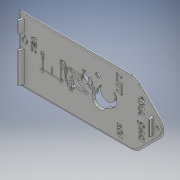
# Autodesk Inventor part: DynamicClampTopCompact
Saved by Autodesk Inventor 2017 (Build 210142000, 142)
## iProperties
Created: 2016-10-04
Part Number: DynamicClampTopCompact
Material: Generic
Document SubType Name: Modeling
Designer: andrew
Density: 1 g/cm^3
Appearance: Default
Author: andrew
Autodesk Inventor part; units mm, degrees
(part 1 of 2)
ref_plane "YZ Plane" through (0, 0, 0) normal (1, 0, 0) x (0, 1, 0)
ref_plane "XZ Plane" through (0, 0, 0) normal (0, 1, 0) x (-1, 0, 0)
ref_plane "XY Plane" through (0, 0, 0) normal (0, 0, 1) x (1, 0, 0)
sketch "Sketch1" plane through (0, 0, 0) normal (0, 1, 0) x (-1, 0, 0)
  line L0 (70.1002, -51.1999) -> (70.1002, -37.9894) construction
  line L1 (70.1002, -37.9894) -> (68.1002, -37.9894) construction
  line L2 (68.1002, -37.9894) -> (68.1002, -48.1999) construction
  arc A0 (67.1002, -49.1999) -> (68.1002, -48.1999) centre (67.1002, -48.1999) ccw construction
  arc A1 (10.6644, -48.6141) -> (12.0787, -49.1999) centre (12.0787, -47.1999) ccw construction
  line L3 (10.6644, -48.6141) -> (10.336, -48.2857) construction
  arc A2 (10.336, -48.2857) -> (8.9218, -47.6999) centre (8.9218, -49.6999) ccw construction
  line L4 (8.9218, -47.6999) -> (-17.9958, -47.6999) construction
  arc A3 (-24.0062, -45.2103) -> (-17.9958, -47.6999) centre (-17.9958, -39.1999) ccw construction
  line L5 (-24.0062, -45.2103) -> (-44.1562, -25.0603) construction
  arc A4 (-44.1562, -13.0395) -> (-44.1562, -25.0603) centre (-38.1458, -19.0499) ccw construction
  line L6 (-44.1562, -13.0395) -> (-24.0062, 7.1105) construction
  arc A5 (-17.9958, 9.6001) -> (-24.0062, 7.1105) centre (-17.9958, 1.1001) ccw construction
  line L7 (-17.9958, 9.6001) -> (8.9218, 9.6001) construction
  arc A6 (8.9218, 9.6001) -> (10.336, 10.1859) centre (8.9218, 11.6001) ccw construction
  line L8 (10.336, 10.1859) -> (10.6644, 10.5143) construction
  arc A7 (12.0787, 11.1001) -> (10.6644, 10.5143) centre (12.0787, 9.1001) ccw construction
  arc A8 (68.1002, 10.1001) -> (67.1002, 11.1001) centre (67.1002, 10.1001) ccw construction
  line L9 (68.1002, 10.1001) -> (68.1002, 5.7045) construction
  line L10 (68.1002, 5.7045) -> (70.1002, 5.7045) construction
  line L11 (70.1002, 5.7045) -> (70.1002, 13.1001) construction
  arc A9 (-17.9958, 13.1001) -> (-26.4811, 9.5854) centre (-17.9958, 1.1001) ccw construction
  line L12 (-26.4811, 9.5854) -> (-46.6311, -10.5646) construction
  arc A10 (-46.6311, -10.5646) -> (-46.6311, -27.5352) centre (-38.1458, -19.0499) ccw construction
  line L13 (-46.6311, -27.5352) -> (-26.4811, -47.6852) construction
  arc A11 (-26.4811, -47.6852) -> (-17.9958, -51.1999) centre (-17.9958, -39.1999) ccw construction
  line L14 (70.1002, -21.9894) -> (70.1002, -6.0043) construction
  line L15 (70.1002, -6.0043) -> (68.1002, -6.0043) construction
  line L16 (68.1002, -6.0043) -> (68.1002, -21.9894) construction
  line L17 (68.1002, -21.9894) -> (70.1002, -21.9894) construction
  line L18 (71.1002, -21.9894) -> (71.1002, -6.0043) construction
  line L19 (71.1002, 5.7045) -> (71.1002, 13.1001) construction
  arc A12 (71.1002, 13.1001) -> (70.1002, 14.1001) centre (70.1002, 13.1001) ccw construction
  arc A13 (-17.9958, 14.1001) -> (-27.1882, 10.2925) centre (-17.9958, 1.1001) ccw construction
  line L20 (-27.1882, 10.2925) -> (-47.3382, -9.8575) construction
  arc A14 (-47.3382, -9.8575) -> (-47.3382, -28.2423) centre (-38.1458, -19.0499) ccw construction
  line L21 (-47.3382, -28.2423) -> (-27.1882, -48.3923) construction
  arc A15 (-27.1882, -48.3923) -> (-17.9958, -52.1999) centre (-17.9958, -39.1999) ccw construction
  arc A16 (70.1002, -52.1999) -> (71.1002, -51.1999) centre (70.1002, -51.1999) ccw construction
  line L22 (71.1002, -51.1999) -> (71.1002, -37.9894) construction
  line L23 (71.1002, -37.9894) -> (70.1002, -37.9894) construction
  line L24 (70.1002, -37.9894) -> (70.1002, -51.1999) construction
  arc A17 (-26.4811, -47.6852) -> (-17.9958, -51.1999) centre (-17.9958, -39.1999) ccw construction
  line L25 (-26.4811, -47.6852) -> (-46.6311, -27.5352) construction
  arc A18 (-46.6311, -10.5646) -> (-46.6311, -27.5352) centre (-38.1458, -19.0499) ccw construction
  line L26 (-46.6311, -10.5646) -> (-26.4811, 9.5854) construction
  arc A19 (-17.9958, 13.1001) -> (-26.4811, 9.5854) centre (-17.9958, 1.1001) ccw construction
  line L27 (70.1002, 13.1001) -> (70.1002, 5.7045) construction
  line L28 (70.1002, 5.7045) -> (71.1002, 5.7045) construction
  line L29 (71.1002, 5.7045) -> (71.1002, 13.1001) construction
  line L30 (71.1002, 5.7045) -> (71.1002, -37.9894) construction
  arc A20 (-44.1562, -13.0395) -> (-44.1562, -25.0603) centre (-38.1458, -19.0499) ccw construction
  line L31 (-46.6458, -19.0499) -> (-58.6779, -19.0499) construction
  arc A21 (-47.3382, -9.8575) -> (-47.3382, -28.2423) centre (-38.1458, -19.0499) ccw construction
  circle A22 centre (-45.0458, -19.0499) radius 1.8
  arc A23 (-23.9239, -50.2423) -> (-14.7316, -54.0499) centre (-14.7316, -41.0499) ccw
  line L32 (-23.9239, -50.2423) -> (-46.6311, -27.5352)
  arc A24 (-46.6311, -10.5646) -> (-46.6311, -27.5352) centre (-38.1458, -19.0499) ccw
  line L33 (-46.6311, -10.5646) -> (-23.9239, 12.1425)
  arc A25 (-14.7316, 15.9501) -> (-23.9239, 12.1425) centre (-14.7316, 2.9501) ccw
  line L34 (109.2514, 15.9501) -> (109.2514, -54.0499)
  arc A26 (-47.3382, -9.8575) -> (-47.3382, -28.2423) centre (-38.1458, -19.0499) ccw
  line L35 (-47.3382, -28.2423) -> (-24.6311, -50.9494)
  arc A27 (-24.6311, -50.9494) -> (-14.7316, -55.0499) centre (-14.7316, -41.0499) ccw
  line L36 (110.2514, -55.0499) -> (110.2514, 16.9501)
  arc A28 (-14.7316, 16.9501) -> (-24.6311, 12.8496) centre (-14.7316, 2.9501) ccw
  line L37 (-24.6311, 12.8496) -> (-47.3382, -9.8575)
  arc A29 (-23.9239, -50.2423) -> (-14.7316, -54.0499) centre (-14.7316, -41.0499) ccw
  line L38 (109.2514, -54.0499) -> (109.2514, 15.9501)
  arc A30 (-14.7316, 15.9501) -> (-23.9239, 12.1425) centre (-14.7316, 2.9501) ccw
  line L39 (-23.9239, 12.1425) -> (-46.6311, -10.5646)
  arc A31 (-46.6311, -10.5646) -> (-46.6311, -27.5352) centre (-38.1458, -19.0499) ccw
  line L40 (-46.6311, -27.5352) -> (-23.9239, -50.2423)
  arc A32 (8.0505, -51.2999) -> (9.3495, -52.0499) centre (9.3495, -50.5499) ccw
  arc A33 (8.0505, -51.2999) -> (6.7514, -50.5499) centre (6.7514, -52.0499) ccw
  line L41 (6.7514, -50.5499) -> (-15.3529, -50.5499)
  arc A34 (-21.0097, -48.2068) -> (-15.3529, -50.5499) centre (-15.3529, -42.5499) ccw
  line L42 (-21.0097, -48.2068) -> (-41.329, -27.8875)
  line L43 (-41.329, -27.8875) -> (-41.329, -10.2123)
  line L44 (-41.329, -10.2123) -> (-21.0097, 10.1069)
  arc A35 (-15.3529, 12.4501) -> (-21.0097, 10.1069) centre (-15.3529, 4.4501) ccw
  line L45 (107.2514, 13.9501) -> (107.2514, -52.0499)
  circle A36 centre (-42.9425, 5.058) radius 1.6
  arc A37 (-47.3382, -9.8575) -> (-47.3382, -28.2423) centre (-38.1458, -19.0499) ccw
  line L46 (-47.3382, -28.2423) -> (-24.6311, -50.9494)
  arc A38 (-24.6311, -50.9494) -> (-14.7316, -55.0499) centre (-14.7316, -41.0499) ccw
  arc A39 (44.182, -57.4874) -> (41.2352, -55.0499) centre (41.2352, -58.0499) ccw
  line L47 (110.2514, -55.0499) -> (110.2514, 16.9501)
  arc A40 (-14.7316, 16.9501) -> (-24.6311, 12.8496) centre (-14.7316, 2.9501) ccw
  line L48 (-24.6311, 12.8496) -> (-47.3382, -9.8575)
  line L49 (71.1002, 32.8345) -> (89.1002, 32.8345)
  line L50 (110.2514, 16.9501) -> (-14.7316, 16.9501)
  line L51 (110.2514, -55.0499) -> (-14.7316, -55.0499)
  point P0 (66.1, 7.6)
  point P1 (-41.329, -19.0499)
  dimension "d177" = 18
  constraints: 104 end point, 79 point on circle, 41 centre point, 2 horizontal, 1 parallel, 1 vertical
  measures "d177" distance of L49.start L49.end
extrude "Extrusion1" add sketch "Sketch1" along normal blind 3 contours L37 A28 L50 L36 L51 A27 L35 A26
sketch "Sketch2" plane through (0, 0, 0) normal (0, -1, 0) x (1, 0, 0)
  circle A0 centre (45.0458, -19.0499) radius 1.8 projected
  line L0 (-110.2514, 16.9501) -> (-110.2514, -55.0499) projected
  line L1 (-110.2514, -55.0499) -> (14.7316, -55.0499) projected
  arc A1 (14.7316, -55.0499) -> (24.6311, -50.9494) centre (14.7316, -41.0499) ccw projected
  line L2 (24.6311, -50.9494) -> (47.3382, -28.2423) projected
  arc A2 (47.3382, -28.2423) -> (47.3382, -9.8575) centre (38.1458, -19.0499) ccw projected
  line L3 (47.3382, -9.8575) -> (24.6311, 12.8496) projected
  arc A3 (24.6311, 12.8496) -> (14.7316, 16.9501) centre (14.7316, 2.9501) ccw projected
  line L4 (14.7316, 16.9501) -> (-110.2514, 16.9501) projected
  line L5 (-108.2514, 14.9501) -> (-108.2514, -53.0499)
  line L6 (-108.2514, -53.0499) -> (14.7316, -53.0499)
  arc A4 (14.7316, -53.0499) -> (23.2168, -49.5352) centre (14.7316, -41.0499) ccw
  line L7 (23.2168, -49.5352) -> (45.9239, -26.8281)
  arc A5 (45.9239, -26.8281) -> (45.9239, -11.2717) centre (38.1458, -19.0499) ccw
  line L8 (45.9239, -11.2717) -> (23.2168, 11.4354)
  arc A6 (23.2168, 11.4354) -> (14.7316, 14.9501) centre (14.7316, 2.9501) ccw
  line L9 (14.7316, 14.9501) -> (-108.2514, 14.9501)
  dimension "d178" = 2
  constraints: 10 end point, 6 point on circle, 3 centre point, 7 other
  measures "d178" distance between parallel lines of L4 L9
extrude "Extrusion2" cut sketch "Sketch2" against normal blind 1 contours L4 A3 L3 A2 L2 A1 L1 L0
fillet "Fillet1" radius 2 8 edges at (20.0891, 3, 15.8844) (35.9846, 3, 1.496) (51.1458, 3, -19.0499) (35.9846, 3, -39.5959) (20.0891, 3, -53.9842) (-47.7599, 3, -55.0499) (-47.7599, 3, 16.9501) (-110.2514, 3, -19.0499)
sketch "Sketch3" plane through (0, 0, 0) normal (0, -1, 0) x (1, 0, 0)
  line L0 (-88.1002, -43.8043) -> (-89.1002, -43.8043) construction
  line L1 (-88.1002, -43.8043) -> (-88.1002, -51.1999) construction
  line L2 (-88.1002, -51.1999) -> (-88.1002, -43.8043) construction
  line L3 (-86.1002, -48.1999) -> (-86.1002, -43.8043) construction
  line L4 (-86.1002, -43.8043) -> (-88.1002, -43.8043) construction
  line L5 (-88.1002, -32.0955) -> (-86.1002, -32.0955) construction
  line L6 (-89.1002, -16.1104) -> (-89.1002, -32.0955) construction
  line L7 (-88.1002, -16.1104) -> (-88.1002, -32.0955) construction
  line L8 (-107.2514, -15.035) -> (-107.2514, 0.9501) construction
  line L9 (-89.1002, -43.8043) -> (-89.1002, -0.1104) construction
  line L10 (-88.1002, -0.1104) -> (-86.1002, -0.1104) construction
  line L11 (-12.0787, -49.1999) -> (-85.1002, -49.1999) construction
  line L12 (-88.1002, -52.1999) -> (17.9958, -52.1999) construction
  line L13 (17.9958, -51.1999) -> (-88.1002, -51.1999) construction
  line L14 (-88.1002, -51.1999) -> (17.9958, -51.1999) construction
  line L15 (-89.1002, -43.8043) -> (-89.1002, -51.1999) construction
  line L16 (-89.1002, -43.8043) -> (-89.1002, -51.1999) construction
  arc A0 (-89.1002, -51.1999) -> (-88.1002, -52.1999) centre (-88.1002, -51.1999) ccw construction
  arc A1 (-86.1002, -48.1999) -> (-85.1002, -49.1999) centre (-85.1002, -48.1999) ccw construction
  line L17 (-89.1002, -0.1104) -> (-88.1002, -0.1104) construction
  line L18 (-10.336, -48.2857) -> (-10.6644, -48.6141) construction
  arc A2 (-8.9218, -47.6999) -> (-10.336, -48.2857) centre (-8.9218, -49.6999) ccw construction
  line L19 (17.9958, -47.6999) -> (-8.9218, -47.6999) construction
  arc A3 (-12.0787, -49.1999) -> (-10.6644, -48.6141) centre (-12.0787, -47.1999) ccw construction
  arc A4 (17.9958, -47.6999) -> (24.0062, -45.2103) centre (17.9958, -39.1999) ccw construction
  arc A5 (17.9958, -51.1999) -> (26.4811, -47.6852) centre (17.9958, -39.1999) ccw construction
  arc A6 (17.9958, -51.1999) -> (26.4811, -47.6852) centre (17.9958, -39.1999) ccw construction
  arc A7 (17.9958, -52.1999) -> (27.1882, -48.3923) centre (17.9958, -39.1999) ccw construction
  line L20 (44.1562, -25.0603) -> (24.0062, -45.2103) construction
  line L21 (41.329, -27.8875) -> (42.2707, -28.8292) construction
  line L22 (41.329, -27.8875) -> (41.329, -10.2123) construction
  line L23 (41.329, -8.1575) -> (41.329, -10.2123) construction
  line L24 (66.5257, -29.0109) -> (68.6689, -29.0109) construction
  line L25 (-106.8514, -19.0499) -> (-106.8514, -34.8081)
  line L26 (-106.8514, -51.1999) -> (-106.8514, -19.0499)
  line L27 (41.329, -27.8875) -> (40.929, -27.8875) construction
  line L28 (40.929, -27.8875) -> (40.929, -27.4875) construction
  line L29 (40.929, -27.4875) -> (38.929, -27.4875) construction
  line L30 (41.329, -10.2123) -> (40.929, -10.2123) construction
  line L31 (40.929, -10.2123) -> (40.929, -10.6123) construction
  line L32 (40.929, -27.4875) -> (40.929, -10.6123)
  line L33 (39.929, -27.4875) -> (39.929, -10.6123)
  line L34 (39.929, -27.4875) -> (40.929, -27.4875)
  line L35 (40.929, -10.6123) -> (39.929, -10.6123)
  line L36 (-105.8514, -19.0499) -> (-105.8514, -51.1999)
  line L37 (-105.8514, -19.0499) -> (-106.8514, -19.0499)
  line L38 (-105.8514, -4.849) -> (-105.8514, -19.0499)
  line L39 (-105.8514, -51.1999) -> (-106.8514, -51.1999)
  line L40 (38.083, 40.4961) -> (20.083, 40.4961)
  point P0 (-84.1, -45.6998)
  point P1 (-18, -38.0998)
  point P2 (-105.8514, -34.8081)
  dimension "d13" = 0.4
  dimension "d14" = 0.4
  dimension "d15" = 2
  dimension "d16" = 0.4
  dimension "d179" = 18
  constraints: 82 end point, 16 point on circle, 8 centre point, 4 perpendicular, 3 horizontal, 3 point on line, 1 collinear, 1 parallel, 1 vertical
  measures "d13" distance of L21.start L27.end
  measures "d14" distance of L27.end L28.end
  measures "d15" distance of L28.end L29.end
  measures "d16" distance of L30.end L31.end
  measures "d179" distance of L40.start L40.end
extrude "Extrusion3" add sketch "Sketch3" along normal blind 5
chamfer "Chamfer1" distance 2 angle 45 1 edges at (46.8458, 3, -19.0499)
chamfer "Chamfer2" distance 2 distance2 5 1 edges at (-105.8514, 0, -35.1249) measured on face at (-25.4628, 0, -19.0499)
chamfer "Chamfer3" distance 2 distance2 5 1 edges at (39.929, 0, -19.0499) measured on face at (-24.7963, 0, -19.0499)
sketch "Sketch15" plane through (0, 3, 0) normal (0, 1, 0) x (1, 0, 0)
  spline S0 degree 4 poles (-27.6915, 13.8507) (-27.1109, 14.9677) (-26.9697, 10.8661) (-22.7238, 18.9014) (-27.3906, 18.904) (-25.9832, 21.4414) knots 0 0 0 0 0 0.383586 1 1 1 1 1
  spline S1 degree 4 poles (-25.9832, 21.4414) (-25.6075, 21.4589) (-25.7778, 23.0598) (-24.46, 21.2542) (-24.2814, 21.5925) (-23.9677, 16.4826) (-23.6468, 16.8653) knots 0 0 0 0 0 0.307527 0.453737 1 1 1 1 1
  spline S2 degree 4 poles (-27.0886, 28.3712) (-27.7683, 25.3166) (-29.1302, 19.4269) (-27.2254, 19.4541) (-27.2142, 16.4527) (-27.0606, 15.6965) (-27.6957, 15.7247) (-28.3997, 16.0175) (-28.7481, 15.0859) (-28.6093, 13.4995) (-27.9401, 12.8786) (-28.544, 10.7453) (-28.3996, 10.1741) (-29.2993, 9.2784) knots 0 0 0 0 0 0.314054 0.389387 0.450233 0.504553 0.55243 0.610485 0.672651 0.739633 0.811347 1 1 1 1 1
  spline S3 degree 4 poles (-23.6468, 16.8653) (-22.0587, 15.4789) (-21.3416, 11.5208) (-19.6026, 10.3039) (-17.2082, 8.3251) knots 0 0 0 0 0 1 1 1 1 1
  arc A0 (-3.9083, 8.3251) -> (-17.2082, 8.3251) centre (-10.5582, 13.1975) ccw
  arc A1 (-3.9083, 8.3251) -> (-5.896, 25.1353) centre (-10.5582, 16.0614) ccw
  spline S4 degree 4 poles (-5.896, 25.1353) (-6.374, 26.5202) (-10.2944, 27.5517) (-11.118, 27.6581) (-15.3167, 32.3371) (-17.6195, 33.2585) (-19.8537, 33.0589) (-22.2655, 32.6919) knots 0 0 0 0 0 0.350642 0.490165 0.626905 1 1 1 1 1
  arc A2 (-22.2655, 32.6919) -> (-27.0886, 28.3712) centre (-20.5674, 25.944) ccw
  spline S5 degree 2 poles (-29.2993, 17.7316) (-28.5886, 18.7822) (-29.3471, 18.5849) knots 0 0 0 1 1 1
  spline S6 degree 3 poles (-29.3471, 18.5849) (-29.4112, 18.5835) (-29.5379, 18.5721) (-29.6879, 18.5392) (-29.8578, 18.486) (-30.0135, 18.4172) (-30.2206, 18.2957) (-30.3804, 18.1742) (-30.5585, 18.0131) (-30.687, 17.8781) (-30.8661, 17.6696) (-31.0304, 17.4539) (-31.2621, 17.1243) (-31.457, 16.8304) (-31.6931, 16.48) (-31.8766, 16.2218) (-32.0734, 15.9767) (-32.1966, 15.845) (-32.3069, 15.7443) (-32.3726, 15.6934) (-32.434, 15.654) (-32.4672, 15.637) (-32.4938, 15.6257) (-32.5083, 15.6207) (-32.523, 15.6167) (-32.5324, 15.6149) (-32.5426, 15.6137) (-32.5502, 15.6134) (-32.5611, 15.6137) (-32.5718, 15.6149) (-32.5892, 15.6182) (-32.6072, 15.6229) (-32.6416, 15.6348) (-32.7013, 15.6611) (-32.7761, 15.7073) (-32.8255, 15.7437) knots 0 0 0 0 0.020676 0.041353 0.051691 0.082705 0.103382 0.144734 0.165411 0.206763 0.22744 0.289469 0.330821 0.413526 0.454879 0.537584 0.578937 0.640966 0.661642 0.702995 0.723671 0.754686 0.765024 0.7857 0.796038 0.816715 0.827053 0.847729 0.858067 0.878744 0.889082 0.909758 0.920096 0.951111 0.992463 0.992463 0.992463 0.992463
  spline S7 degree 3 poles (-33.3316, 15.0565) (-31.4073, 13.6393) (-30.5877, 17.7655) (-29.2993, 17.7316) knots 0 0 0 0 1 1 1 1
  spline S8 degree 3 poles (-29.2993, 9.2784) (-28.4253, 9.2006) (-27.1186, 12.6954) (-27.6915, 13.8507) knots 0 0 0 0 1 1 1 1
  spline S9 degree 2 poles (-29.8702, 7.4447) (-28.4119, 7.7455) (-29.3465, 8.5308) knots 0 0 0 1 1 1
  arc A3 (-32.8397, 9.4959) -> (-33.3316, 15.0565) centre (-36.3694, 11.9857) ccw
  spline S10 degree 3 poles (-29.3465, 8.5308) (-30.3224, 8.9378) (-31.6097, 9.7155) (-32.8397, 9.4959) knots 0 0 0 0 1 1 1 1
  spline S11 degree 3 poles (-32.4084, 8.33) (-32.3583, 8.3304) (-32.2532, 8.3264) (-32.1091, 8.3083) (-31.9561, 8.2801) (-31.8271, 8.2495) (-31.6588, 8.2018) (-31.5192, 8.1564) (-31.3397, 8.0916) (-31.1926, 8.0339) (-31.0054, 7.9559) (-30.8534, 7.8894) (-30.6228, 7.7854) (-30.3112, 7.641) (-30.033, 7.514) (-29.8702, 7.4447) knots 0.113605 0.113605 0.113605 0.113605 0.185987 0.258369 0.29456 0.366942 0.403132 0.475514 0.511705 0.584087 0.620278 0.69266 0.72885 0.837423 0.982187 0.982187 0.982187 0.982187
  spline S12 degree 2 poles (-34.4115, 8.1354) (-33.303, 7.9123) (-32.4084, 8.33) knots 0 0 0 1 1 1
  spline S13 degree 4 poles (-56.5582, 22.2724) (-56.0745, 22.1932) (-55.5294, 22.4303) (-55.1686, 23.657) (-55.4245, 24.7118) (-55.684, 26.6227) (-55.267, 27.7234) (-54.7915, 28.7982) knots 1 1 1 1 1 2 3 4 5 5 5 5 5
  spline S14 degree 4 poles (-54.7915, 28.7982) (-55.8528, 27.8241) (-56.4014, 26.069) (-56.3468, 24.2397) (-56.6058, 23.8256) (-56.9416, 24.0302) knots 1 1 1 1 1 2 3 3 3 3 3
  spline S15 degree 4 poles (-56.9416, 24.0302) (-56.9765, 24.0427) (-57.1392, 24.138) (-57.4252, 24.5671) (-58.0911, 25.0409) (-58.5876, 23.2825) (-58.4587, 21.8862) (-58.4587, 18.1761) (-58.8463, 14.3452) (-59.8927, 11.0836) (-61.104, 9.7327) (-62.5294, 9.0563) (-63.199, 10.049) (-63.0001, 11.4417) (-62.3618, 12.4482) (-62.053, 13.8507) (-61.4936, 14.3452) (-60.8562, 14.7607) (-61.4832, 15.3588) (-61.987, 15.6025) (-62.2074, 15.6753) knots 21.225328 21.225328 21.225328 21.225328 21.225328 21.495604 22.495604 23.495604 24.495604 25.495604 26.495604 27.495604 28.495604 29.495604 30.495604 31.495604 32.495604 33.495604 34.495604 35.495604 36.495604 37.270276 37.270276 37.270276 37.270276 37.270276
  spline S16 degree 4 poles (-63.0718, 15.7424) (-63.1596, 15.7216) (-63.4415, 15.619) (-63.7505, 15.2916) (-63.7505, 14.8717) (-62.9882, 14.4366) (-62.9882, 13.7604) (-62.9882, 12.3663) (-63.9484, 11.3247) (-64.2146, 9.4959) (-63.6303, 7.3568) (-62.5708, 6.4807) (-59.9153, 6.0705) (-56.4013, 8.7612) (-55.5617, 14.6392) (-56.6999, 19.159) (-57.2516, 21.4603) (-56.8901, 22.1314) (-56.6535, 22.255) (-56.5582, 22.2724) knots 5.292479 5.292479 5.292479 5.292479 5.292479 5.692476 6.692476 7.692476 8.692476 9.692476 10.692476 11.692476 12.692476 13.692476 14.692476 15.692476 16.692476 17.692476 18.692476 19.692476 20.399997 20.399997 20.399997 20.399997 20.399997
  line L0 (-62.2074, 15.6753) -> (-62.2074, 26.2032)
  line L1 (-63.0001, 26.2148) -> (-63.0718, 15.7424)
  line L2 (-61.4936, 25.1069) -> (-60.2137, 26.59)
  line L3 (-62.2074, 26.2032) -> (-61.4936, 25.1069)
  line L4 (-60.2137, 26.59) -> (-63.0001, 29.7217)
  line L5 (-63.0001, 29.7217) -> (-64.5425, 28.3494)
  line L6 (-72.4079, 26.2793) -> (-63.0001, 26.2148)
  spline S17 degree 2 poles (-32.8255, 15.7437) (-33.3769, 15.7671) (-34.1345, 15.682) knots 0 0 0 1 1 1
  arc A4 (-34.1345, 15.682) -> (-40.0719, 14.2105) centre (-36.3694, 11.9857) ccw
  spline S18 degree 4 poles (-53.9061, 12.1086) (-54.7915, 11.4417) (-54.962, 10.4932) (-54.3382, 9.4959) (-52.9763, 9.3945) (-49.6794, 9.4959) (-45.0315, 10.0217) (-42.8113, 10.0472) (-41.7631, 10.0046) (-41.3306, 9.9364) knots 1 1 1 1 1 2 3 4 5 6 6.802438 6.802438 6.802438 6.802438 6.802438
  spline S19 degree 2 poles (-41.1494, 14.9301) (-40.4153, 14.9287) (-40.5797, 12.951) knots 0 0 0 1 1 1
  spline S20 degree 4 poles (-40.0719, 14.2105) (-40.9135, 16.1942) (-39.8855, 15.3008) (-43.4443, 17.9593) (-44.4211, 13.9055) (-42.0945, 15.658) (-42.243, 15.1104) (-41.1494, 14.9301) knots 0 0 0 0 0 0.398573 0.540898 0.679309 1 1 1 1 1
  arc A5 (-40.5797, 12.951) -> (-40.6887, 11.939) centre (-36.3694, 11.9857) ccw
  spline S21 degree 3 poles (-40.6887, 11.939) (-44.5291, 12.1277) (-45.5557, 11.7883) (-52.4316, 11.4417) knots 0 0 0 0 1 1 1 1
  line L7 (-46.08, 23.8106) -> (-34.4115, 24.2928)
  line L8 (-33.3316, 25.944) -> (-46.1463, 25.4145)
  spline S22 degree 2 poles (-32.6574, 23.8106) (-32.3348, 24.8678) (-33.3316, 25.944) knots 0 0 0 1 1 1
  line L9 (-34.4115, 24.2928) -> (-53.9061, 12.1086)
  line L10 (-52.4316, 11.4417) -> (-32.6574, 23.8106)
  spline S23 degree 4 poles (-46.1463, 25.4145) (-46.9929, 25.944) (-48.4992, 27.7972) (-49.6125, 28.1943) (-49.3506, 30.0281) (-50.6059, 32.035) (-51.694, 31.3544) (-50.9878, 29.7661) (-50.9878, 28.6547) (-52.2322, 29.4387) (-53.1194, 30.8571) (-52.1667, 32.5347) (-54.0032, 30.4865) (-54.0032, 29.3042) (-52.4316, 27.7972) (-51.7737, 27.2775) (-50.9878, 26.8502) (-53.1403, 26.8502) (-54.6732, 25.944) (-54.0032, 24.4613) (-53.2302, 24.829) (-53.2302, 25.4145) (-51.9702, 25.944) (-50.9224, 25.4145) (-50.4532, 24.6645) (-51.5773, 23.2825) (-53.6006, 23.2825) (-54.3308, 22.091) (-52.8216, 21.8417) (-50.9224, 22.6276) (-50.9224, 21.1449) (-52.9164, 19.8976) (-54.0032, 19.2681) (-53.1534, 18.068) (-51.7312, 18.9852) (-50.9224, 19.8769) (-51.5118, 16.8688) (-50.0738, 15.682) (-49.809, 16.8688) (-50.0738, 18.4598) (-49.2851, 19.2875) (-48.2372, 20.7283) (-48.4992, 22.141) (-47.3858, 24.829) (-46.08, 23.8106) knots 1 1 1 1 1 2 3 4 5 6 7 8 9 10 11 12 13 14 15 16 17 18 19 20 21 22 23 24 25 26 27 28 29 30 31 32 33 34 35 36 37 38 39 40 41 42 42 42 42 42
  line L11 (-83.291, 16.3362) -> (-83.0145, 17.7316)
  line L12 (-83.291, 17.8877) -> (-84.6947, 15.6753)
  line L13 (-81.7763, 15.9699) -> (-83.291, 16.3362)
  line L14 (-84.6947, 15.6753) -> (-83.291, 15.6753)
  line L15 (-82.7096, 13.4874) -> (-81.7763, 15.9699)
  line L16 (-81.2462, 13.4874) -> (-82.7096, 13.4874)
  line L17 (-83.291, 15.6753) -> (-85.644, 12.3663)
  line L18 (-85.644, 12.3663) -> (-83.6731, 12.3663)
  line L19 (-85.644, 9.5946) -> (-82.7096, 9.5946)
  line L20 (-83.6731, 12.3663) -> (-85.644, 9.5946)
  line L21 (-82.7096, 9.5946) -> (-81.2462, 13.4874)
  line L22 (-64.5425, 28.3494) -> (-63.4286, 27.0974)
  line L23 (-63.4286, 27.0974) -> (-83.4506, 27.0974)
  line L24 (-83.4506, 27.0974) -> (-82.0904, 28.5507)
  line L25 (-83.8017, 18.1761) -> (-83.291, 17.8877)
  line L26 (-73.4396, 19.6918) -> (-72.4541, 19.5315)
  line L27 (-83.0145, 17.7316) -> (-82.9554, 26.3515)
  line L28 (-83.8017, 26.7223) -> (-83.8017, 18.1761)
  line L29 (-84.847, 25.6055) -> (-83.8017, 26.7223)
  line L30 (-86.441, 27.0974) -> (-84.847, 25.6055)
  line L31 (-83.291, 29.9001) -> (-86.441, 27.0974)
  line L32 (-82.0904, 28.5507) -> (-83.291, 29.9001)
  line L33 (-82.9554, 26.3515) -> (-73.4396, 26.2863)
  line L34 (-72.4541, 19.5315) -> (-72.4079, 26.2793)
  line L35 (-73.4396, 26.2863) -> (-73.4396, 19.6918)
  arc A6 (-37.1649, 7.7401) -> (-34.4115, 8.1354) centre (-36.3694, 11.9857) ccw
  spline S24 degree 4 poles (-41.3306, 9.9364) (-41.2242, 9.9196) (-40.5914, 9.7998) (-40.0125, 9.5498) (-39.3261, 9.0075) (-38.1511, 8.0507) knots 6.802438 6.802438 6.802438 6.802438 6.802438 7 8 8 8 8 8
  spline S25 degree 3 poles (-38.1511, 8.0507) (-37.8088, 6.7326) (-37.6644, 4.2869) (-38.5809, 4.7262) knots 0 0 0 0 1 1 1 1
  spline S26 degree 4 poles (-36.4347, 4.1098) (-36.8593, 3.1985) (-34.0229, 2.8853) (-35.3987, 5.2081) (-37.4947, 5.1686) (-36.4212, 6.3109) (-37.0004, 7.6075) (-37.1649, 7.7401) knots 0 0 0 0 0 0.379017 0.523779 0.680013 0.97265 0.97265 0.97265 0.97265 0.97265
  spline S27 degree 4 poles (-38.5809, 4.7262) (-38.9921, 5.2003) (-40.1563, 4.7172) (-38.3235, 2.8066) (-37.8223, 5.0385) (-36.2931, 4.6806) (-36.4347, 4.1098) knots 0 0 0 0 0 0.393852 0.564941 1 1 1 1 1
  spline S28 degree 4 poles (-27.6915, 13.8507) (-27.1109, 14.9677) (-26.9697, 10.8661) (-22.7238, 18.9014) (-27.3906, 18.904) (-25.9832, 21.4414) knots 0 0 0 0 0 0.383586 1 1 1 1 1
  spline S29 degree 4 poles (-25.9832, 21.4414) (-25.6075, 21.4589) (-25.7778, 23.0598) (-24.46, 21.2542) (-24.2814, 21.5925) (-23.9677, 16.4826) (-23.6468, 16.8653) knots 0 0 0 0 0 0.307527 0.453737 1 1 1 1 1
  spline S30 degree 4 poles (-27.0886, 28.3712) (-27.7683, 25.3166) (-29.1302, 19.4269) (-27.2254, 19.4541) (-27.2142, 16.4527) (-27.0606, 15.6965) (-27.6957, 15.7247) (-28.3997, 16.0175) (-28.7481, 15.0859) (-28.6093, 13.4995) (-27.9401, 12.8786) (-28.544, 10.7453) (-28.3996, 10.1741) (-29.2993, 9.2784) knots 0 0 0 0 0 0.314054 0.389387 0.450233 0.504553 0.55243 0.610485 0.672651 0.739633 0.811347 1 1 1 1 1
  spline S31 degree 4 poles (-23.6468, 16.8653) (-22.0587, 15.4789) (-21.3416, 11.5208) (-19.6026, 10.3039) (-17.2082, 8.3251) knots 0 0 0 0 0 1 1 1 1 1
  arc A7 (-3.9083, 8.3251) -> (-17.2082, 8.3251) centre (-10.5582, 13.1975) ccw
  arc A8 (-3.9083, 8.3251) -> (-5.896, 25.1353) centre (-10.5582, 16.0614) ccw
  spline S32 degree 4 poles (-5.896, 25.1353) (-6.374, 26.5202) (-10.2944, 27.5517) (-11.118, 27.6581) (-15.3167, 32.3371) (-17.6195, 33.2585) (-19.8537, 33.0589) (-22.2655, 32.6919) knots 0 0 0 0 0 0.350642 0.490165 0.626905 1 1 1 1 1
  arc A9 (-22.2655, 32.6919) -> (-27.0886, 28.3712) centre (-20.5674, 25.944) ccw
  spline S33 degree 2 poles (-29.2993, 17.7316) (-28.5886, 18.7822) (-29.3471, 18.5849) knots 0 0 0 1 1 1
  spline S34 degree 3 poles (-29.3471, 18.5849) (-29.4112, 18.5835) (-29.5379, 18.5721) (-29.6879, 18.5392) (-29.8578, 18.486) (-30.0135, 18.4172) (-30.2206, 18.2957) (-30.3804, 18.1742) (-30.5585, 18.0131) (-30.687, 17.8781) (-30.8661, 17.6696) (-31.0304, 17.4539) (-31.2621, 17.1243) (-31.457, 16.8304) (-31.6931, 16.48) (-31.8766, 16.2218) (-32.0734, 15.9767) (-32.1966, 15.845) (-32.3069, 15.7443) (-32.3726, 15.6934) (-32.434, 15.654) (-32.4672, 15.637) (-32.4938, 15.6257) (-32.5083, 15.6207) (-32.523, 15.6167) (-32.5324, 15.6149) (-32.5426, 15.6137) (-32.5502, 15.6134) (-32.5611, 15.6137) (-32.5718, 15.6149) (-32.5892, 15.6182) (-32.6072, 15.6229) (-32.6416, 15.6348) (-32.7013, 15.6611) (-32.7761, 15.7073) (-32.8255, 15.7437) knots 0 0 0 0 0.020676 0.041353 0.051691 0.082705 0.103382 0.144734 0.165411 0.206763 0.22744 0.289469 0.330821 0.413526 0.454879 0.537584 0.578937 0.640966 0.661642 0.702995 0.723671 0.754686 0.765024 0.7857 0.796038 0.816715 0.827053 0.847729 0.858067 0.878744 0.889082 0.909758 0.920096 0.951111 0.992463 0.992463 0.992463 0.992463
  spline S35 degree 3 poles (-33.3316, 15.0565) (-31.4073, 13.6393) (-30.5877, 17.7655) (-29.2993, 17.7316) knots 0 0 0 0 1 1 1 1
  spline S36 degree 3 poles (-29.2993, 9.2784) (-28.4253, 9.2006) (-27.1186, 12.6954) (-27.6915, 13.8507) knots 0 0 0 0 1 1 1 1
  spline S37 degree 2 poles (-29.8702, 7.4447) (-28.4119, 7.7455) (-29.3465, 8.5308) knots 0 0 0 1 1 1
  arc A10 (-32.8397, 9.4959) -> (-33.3316, 15.0565) centre (-36.3694, 11.9857) ccw
  spline S38 degree 3 poles (-29.3465, 8.5308) (-30.3224, 8.9378) (-31.6097, 9.7155) (-32.8397, 9.4959) knots 0 0 0 0 1 1 1 1
  spline S39 degree 3 poles (-32.4084, 8.33) (-32.3583, 8.3304) (-32.2532, 8.3264) (-32.1091, 8.3083) (-31.9561, 8.2801) (-31.8271, 8.2495) (-31.6588, 8.2018) (-31.5192, 8.1564) (-31.3397, 8.0916) (-31.1926, 8.0339) (-31.0054, 7.9559) (-30.8534, 7.8894) (-30.6228, 7.7854) (-30.3112, 7.641) (-30.033, 7.514) (-29.8702, 7.4447) knots 0.113605 0.113605 0.113605 0.113605 0.185987 0.258369 0.29456 0.366942 0.403132 0.475514 0.511705 0.584087 0.620278 0.69266 0.72885 0.837423 0.982187 0.982187 0.982187 0.982187
  spline S40 degree 2 poles (-34.4115, 8.1354) (-33.303, 7.9123) (-32.4084, 8.33) knots 0 0 0 1 1 1
  spline S41 degree 4 poles (-56.5582, 22.2724) (-56.0745, 22.1932) (-55.5294, 22.4303) (-55.1686, 23.657) (-55.4245, 24.7118) (-55.684, 26.6227) (-55.267, 27.7234) (-54.7915, 28.7982) knots 1 1 1 1 1 2 3 4 5 5 5 5 5
  spline S42 degree 4 poles (-54.7915, 28.7982) (-55.8528, 27.8241) (-56.4014, 26.069) (-56.3468, 24.2397) (-56.6058, 23.8256) (-56.9416, 24.0302) knots 1 1 1 1 1 2 3 3 3 3 3
  spline S43 degree 4 poles (-56.9416, 24.0302) (-56.9765, 24.0427) (-57.1392, 24.138) (-57.4252, 24.5671) (-58.0911, 25.0409) (-58.5876, 23.2825) (-58.4587, 21.8862) (-58.4587, 18.1761) (-58.8463, 14.3452) (-59.8927, 11.0836) (-61.104, 9.7327) (-62.5294, 9.0563) (-63.199, 10.049) (-63.0001, 11.4417) (-62.3618, 12.4482) (-62.053, 13.8507) (-61.4936, 14.3452) (-60.8562, 14.7607) (-61.4832, 15.3588) (-61.987, 15.6025) (-62.2074, 15.6753) knots 21.225328 21.225328 21.225328 21.225328 21.225328 21.495604 22.495604 23.495604 24.495604 25.495604 26.495604 27.495604 28.495604 29.495604 30.495604 31.495604 32.495604 33.495604 34.495604 35.495604 36.495604 37.270276 37.270276 37.270276 37.270276 37.270276
  spline S44 degree 4 poles (-63.0718, 15.7424) (-63.1596, 15.7216) (-63.4415, 15.619) (-63.7505, 15.2916) (-63.7505, 14.8717) (-62.9882, 14.4366) (-62.9882, 13.7604) (-62.9882, 12.3663) (-63.9484, 11.3247) (-64.2146, 9.4959) (-63.6303, 7.3568) (-62.5708, 6.4807) (-59.9153, 6.0705) (-56.4013, 8.7612) (-55.5617, 14.6392) (-56.6999, 19.159) (-57.2516, 21.4603) (-56.8901, 22.1314) (-56.6535, 22.255) (-56.5582, 22.2724) knots 5.292479 5.292479 5.292479 5.292479 5.292479 5.692476 6.692476 7.692476 8.692476 9.692476 10.692476 11.692476 12.692476 13.692476 14.692476 15.692476 16.692476 17.692476 18.692476 19.692476 20.399997 20.399997 20.399997 20.399997 20.399997
  line L36 (-62.2074, 15.6753) -> (-62.2074, 26.2032)
  line L37 (-63.0001, 26.2148) -> (-63.0718, 15.7424)
  line L38 (-61.4936, 25.1069) -> (-60.2137, 26.59)
  line L39 (-62.2074, 26.2032) -> (-61.4936, 25.1069)
  line L40 (-60.2137, 26.59) -> (-63.0001, 29.7217)
  line L41 (-63.0001, 29.7217) -> (-64.5425, 28.3494)
  line L42 (-72.4079, 26.2793) -> (-63.0001, 26.2148)
  spline S45 degree 2 poles (-32.8255, 15.7437) (-33.3769, 15.7671) (-34.1345, 15.682) knots 0 0 0 1 1 1
  arc A11 (-34.1345, 15.682) -> (-40.0719, 14.2105) centre (-36.3694, 11.9857) ccw
  spline S46 degree 4 poles (-53.9061, 12.1086) (-54.7915, 11.4417) (-54.962, 10.4932) (-54.3382, 9.4959) (-52.9763, 9.3945) (-49.6794, 9.4959) (-45.0315, 10.0217) (-42.8113, 10.0472) (-41.7631, 10.0046) (-41.3306, 9.9364) knots 1 1 1 1 1 2 3 4 5 6 6.802438 6.802438 6.802438 6.802438 6.802438
  spline S47 degree 2 poles (-41.1494, 14.9301) (-40.4153, 14.9287) (-40.5797, 12.951) knots 0 0 0 1 1 1
  spline S48 degree 4 poles (-40.0719, 14.2105) (-40.9135, 16.1942) (-39.8855, 15.3008) (-43.4443, 17.9593) (-44.4211, 13.9055) (-42.0945, 15.658) (-42.243, 15.1104) (-41.1494, 14.9301) knots 0 0 0 0 0 0.398573 0.540898 0.679309 1 1 1 1 1
  arc A12 (-40.5797, 12.951) -> (-40.6887, 11.939) centre (-36.3694, 11.9857) ccw
  spline S49 degree 3 poles (-40.6887, 11.939) (-44.5291, 12.1277) (-45.5557, 11.7883) (-52.4316, 11.4417) knots 0 0 0 0 1 1 1 1
  line L43 (-46.08, 23.8106) -> (-34.4115, 24.2928)
  line L44 (-33.3316, 25.944) -> (-46.1463, 25.4145)
  spline S50 degree 2 poles (-32.6574, 23.8106) (-32.3348, 24.8678) (-33.3316, 25.944) knots 0 0 0 1 1 1
  line L45 (-34.4115, 24.2928) -> (-53.9061, 12.1086)
  line L46 (-52.4316, 11.4417) -> (-32.6574, 23.8106)
  spline S51 degree 4 poles (-46.1463, 25.4145) (-46.9929, 25.944) (-48.4992, 27.7972) (-49.6125, 28.1943) (-49.3506, 30.0281) (-50.6059, 32.035) (-51.694, 31.3544) (-50.9878, 29.7661) (-50.9878, 28.6547) (-52.2322, 29.4387) (-53.1194, 30.8571) (-52.1667, 32.5347) (-54.0032, 30.4865) (-54.0032, 29.3042) (-52.4316, 27.7972) (-51.7737, 27.2775) (-50.9878, 26.8502) (-53.1403, 26.8502) (-54.6732, 25.944) (-54.0032, 24.4613) (-53.2302, 24.829) (-53.2302, 25.4145) (-51.9702, 25.944) (-50.9224, 25.4145) (-50.4532, 24.6645) (-51.5773, 23.2825) (-53.6006, 23.2825) (-54.3308, 22.091) (-52.8216, 21.8417) (-50.9224, 22.6276) (-50.9224, 21.1449) (-52.9164, 19.8976) (-54.0032, 19.2681) (-53.1534, 18.068) (-51.7312, 18.9852) (-50.9224, 19.8769) (-51.5118, 16.8688) (-50.0738, 15.682) (-49.809, 16.8688) (-50.0738, 18.4598) (-49.2851, 19.2875) (-48.2372, 20.7283) (-48.4992, 22.141) (-47.3858, 24.829) (-46.08, 23.8106) knots 1 1 1 1 1 2 3 4 5 6 7 8 9 10 11 12 13 14 15 16 17 18 19 20 21 22 23 24 25 26 27 28 29 30 31 32 33 34 35 36 37 38 39 40 41 42 42 42 42 42
  line L47 (-83.291, 16.3362) -> (-83.0145, 17.7316)
  line L48 (-83.291, 17.8877) -> (-84.6947, 15.6753)
  line L49 (-81.7763, 15.9699) -> (-83.291, 16.3362)
  line L50 (-84.6947, 15.6753) -> (-83.291, 15.6753)
  line L51 (-82.7096, 13.4874) -> (-81.7763, 15.9699)
  line L52 (-81.2462, 13.4874) -> (-82.7096, 13.4874)
  line L53 (-83.291, 15.6753) -> (-85.644, 12.3663)
  line L54 (-85.644, 12.3663) -> (-83.6731, 12.3663)
  line L55 (-85.644, 9.5946) -> (-82.7096, 9.5946)
  line L56 (-83.6731, 12.3663) -> (-85.644, 9.5946)
  line L57 (-82.7096, 9.5946) -> (-81.2462, 13.4874)
  line L58 (-64.5425, 28.3494) -> (-63.4286, 27.0974)
  line L59 (-63.4286, 27.0974) -> (-83.4506, 27.0974)
  line L60 (-83.4506, 27.0974) -> (-82.0904, 28.5507)
  line L61 (-83.8017, 18.1761) -> (-83.291, 17.8877)
  line L62 (-73.4396, 19.6918) -> (-72.4541, 19.5315)
  line L63 (-83.0145, 17.7316) -> (-82.9554, 26.3515)
  line L64 (-83.8017, 26.7223) -> (-83.8017, 18.1761)
  line L65 (-84.847, 25.6055) -> (-83.8017, 26.7223)
  line L66 (-86.441, 27.0974) -> (-84.847, 25.6055)
  line L67 (-83.291, 29.9001) -> (-86.441, 27.0974)
  line L68 (-82.0904, 28.5507) -> (-83.291, 29.9001)
  line L69 (-82.9554, 26.3515) -> (-73.4396, 26.2863)
  line L70 (-72.4541, 19.5315) -> (-72.4079, 26.2793)
  line L71 (-73.4396, 26.2863) -> (-73.4396, 19.6918)
  arc A13 (-37.1649, 7.7401) -> (-34.4115, 8.1354) centre (-36.3694, 11.9857) ccw
  spline S52 degree 4 poles (-41.3306, 9.9364) (-41.2242, 9.9196) (-40.5914, 9.7998) (-40.0125, 9.5498) (-39.3261, 9.0075) (-38.1511, 8.0507) knots 6.802438 6.802438 6.802438 6.802438 6.802438 7 8 8 8 8 8
  spline S53 degree 3 poles (-38.1511, 8.0507) (-37.8088, 6.7326) (-37.6644, 4.2869) (-38.5809, 4.7262) knots 0 0 0 0 1 1 1 1
  spline S54 degree 4 poles (-36.4347, 4.1098) (-36.8593, 3.1985) (-34.0229, 2.8853) (-35.3987, 5.2081) (-37.4947, 5.1686) (-36.4212, 6.3109) (-37.0004, 7.6075) (-37.1649, 7.7401) knots 0 0 0 0 0 0.379017 0.523779 0.680013 0.97265 0.97265 0.97265 0.97265 0.97265
  spline S55 degree 4 poles (-38.5809, 4.7262) (-38.9921, 5.2003) (-40.1563, 4.7172) (-38.3235, 2.8066) (-37.8223, 5.0385) (-36.2931, 4.6806) (-36.4347, 4.1098) knots 0 0 0 0 0 0.393852 0.564941 1 1 1 1 1
  point P0 (-73.6712, 53.4504)
  constraints: 144 end point, 28 point on circle, 14 centre point, 154 other
extrude "Extrusion14" cut sketch "Sketch15" against normal blind 10
sketch "Sketch17" plane through (-106.8514, -5, -19.0499) normal (0, 0, 1) x (1, 0, 0)
  line L0 (147.7804, 5) -> (147.7804, 0) projected
  line L1 (147.7804, 0) -> (146.7804, 0) projected
  line L2 (147.7804, 0.5357) -> (147.7804, 2) projected
  line L3 (147.7804, 0.5357) -> (148.6804, 1.5) projected
  line L4 (148.6804, 1.5) -> (148.6804, 2) projected
  line L5 (148.6804, 2) -> (147.7804, 2) projected
  line L6 (147.7804, 0) -> (146.7804, 0) projected
  line L7 (0, 0) -> (1, 0) projected
  line L8 (146.7804, 0) -> (1, 0)
  line L9 (73.8902, 0) -> (73.8902, -91.1648)
  line L10 (0.5, 0) -> (0, 0.5357)
  line L11 (0, 5) -> (0, 0.5357)
  line L12 (3, 5) -> (0, 5)
  line L13 (1, 0) -> (3, 5)
  line L14 (0.5, 0) -> (1, 0)
  line L15 (0, 0.5357) -> (0, 2)
  line L16 (0, 0.5357) -> (-0.9, 1.5)
  line L17 (-0.9, 1.5) -> (-0.9, 2)
  line L18 (-0.9, 2) -> (0, 2)
  line L19 (0.5, 0) -> (1, 0)
  line L20 (1, 0) -> (146.7804, 0)
  line L21 (144.7804, 5) -> (147.7804, 5) projected
  line L22 (146.7804, 0) -> (144.7804, 5) projected
  point P0 (106.8514, 5)
  point P1 (147.2804, 0)
  constraints: 26 end point, 6 symmetric about line, 1 horizontal, 1 midpoint, 1 vertical
extrude "Extrusion15" add sketch "Sketch17" against normal blind 32.15 contours L16 L17 L18 L11
sketch "Sketch18" plane through (-103.8514, 0, -51.1999) normal (0, 0, -1) x (-1, 0, 0)
  line L0 (3.9, -3.5) -> (3, -4.4643) construction
  line L1 (3, -4.4643) -> (3.9, -3.5) construction
  line L2 (3.9, -3.5) -> (3.9, -5.7276) construction
  line L3 (3.9, -5.7276) -> (1.5224, -5.7276) construction
  line L4 (3, 0) -> (3, -5) construction
  line L5 (3, -4.4643) -> (1.8209, -5.7276) construction
  line L6 (3.9, -3.5) -> (1.8209, -5.7276)
  line L7 (1.8209, -5.7276) -> (3.9, -5.7276)
  line L8 (3.9, -5.7276) -> (3.9, -3.5)
  point P0 (-103.8514, 0)
  point P1 (21, -4.4643)
  constraints: 14 end point, 2 vertical, 1 horizontal, 1 perpendicular, 2 other
extrude "Extrusion16" cut sketch "Sketch18" against normal blind 40